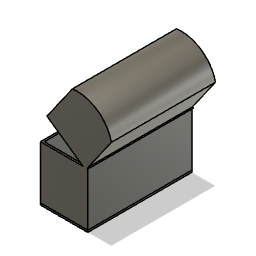
Shape 5 (Autodesk Fusion 360 design; units mm, degrees)
Autodesk Fusion 360 part; units mm, degrees
note: some values were not read from the file. Chosen so that the rebuilt part matches the saved one: which bodies a step acts on.
sketch "Sketch1" plane through (0, 0, 0) normal (0, 1, 0) x (1, 0, 0)
  line L0 (-25, 25) -> (0, 25)
  line L1 (0, 25) -> (0, -30)
  line L2 (0, -30) -> (-25, -30)
  line L3 (-25, -30) -> (-25, 25)
  constraint horizontal L0
  constraint vertical L1
  constraint horizontal L2
  constraint vertical L3
extrude "Extrude1" add sketch "Sketch1" along normal blind 50 makes body 1
sketch "Sketch2" plane through (0, 0, 0) normal (0, 0, 1) x (1, 0, 0)
  circle A0 centre (-12.3509, 42.7444) radius 18.4875
extrude "Extrude2" add sketch "Sketch2" along normal blind 30 and the other way blind 25 bodies 1
sketch "Sketch3" plane through (0, 0, 0) normal (0, 0, 1) x (1, 0, 0)
  line L0 (0, 30) -> (20, 30)
  line L1 (20, 30) -> (20, 60)
  line L2 (20, 60) -> (0, 60)
  line L3 (0, 60) -> (0, 30)
  line L4 (-25, 30) -> (-40, 30)
  line L5 (-40, 30) -> (-40, 60)
  line L6 (-40, 60) -> (-25, 60)
  line L7 (-25, 60) -> (-25, 30)
  constraint horizontal L0
  constraint vertical L1
  constraint horizontal L2
  constraint vertical L3
  constraint horizontal L4
  constraint vertical L5
  constraint horizontal L6
  constraint vertical L7
extrude "Extrude3" cut sketch "Sketch3" along normal blind 45 and the other way blind 55 bodies 1
sketch "Sketch4" plane through (0, 0, 0) normal (0, 1, 0) x (1, 0, 0)
  line L0 (-30, 25) -> (5, 25)
  line L1 (5, 25) -> (5, -35)
  line L2 (5, -35) -> (-30, -35)
  line L3 (-30, -35) -> (-30, 25)
  constraint horizontal L0
  constraint vertical L1
  constraint horizontal L2
  constraint vertical L3
extrude "Extrude4" add sketch "Sketch4" along normal blind 1 separate body makes body 2
split "Split1" by bodies 2 bodies 1 makes body 3 at (-25, 19.8411, 11.6667)
move_body "Move1" bodies 2 to x (1, 0, 0) y (0, 1, 0) z (0, 0, 1) at (0, 30, 0)
split "Split2" by bodies 2 bodies 3 makes body 4 at (-25, 19.8411, 11.6667) makes body 5 at (-23.6053, 57.4116, 11.6667)
move_body "Move2" bodies 5 to x (0.707107, -0.707107, 0) y (0.707107, 0.707107, 0) z (0, 0, 1) at (-20.9275, 9.171, 0)
shell "Shell1" thickness 1 removed faces 0 bodies 5
move_body "Move3" bodies 5 to x (1, 0, 0) y (0, 1, 0) z (0, 0, 1) at (-3.5355, -3.5355, 0)
sketch "Sketch5" plane through (0, 0, 0) normal (0, 1, 0) x (1, 0, 0)
  line L0 (-30, 25) -> (0, 25)
  line L1 (0, 25) -> (0, -35)
  line L2 (0, -35) -> (-30, -35)
  line L3 (-30, -35) -> (-30, 25)
  constraint horizontal L0
  constraint vertical L1
  constraint horizontal L2
  constraint vertical L3
shell "Shell2" thickness 1 removed faces 0 bodies 4
extrude "Extrude5" add sketch "Sketch5" along normal blind 2 separate body makes body 6
move_body "Move4" bodies 6 to x (1, 0, 0) y (0, 1, 0) z (0, 0, 1) at (0, 29, 0)
split "Split3" by bodies 6 bodies 4 makes body 7 at (-25, 19.6667, 11.6667)
move_body "Move5" bodies 5 to x (0.707107, 0.707107, 0) y (-0.707107, 0.707107, 0) z (0, 0, 1) at (64.1238, 37.9942, 0)
sketch "Sketch6" plane through (0, 0, 0) normal (0, 1, 0) x (1, 0, 0)
  line L0 (15, 30) -> (45, 30)
  line L1 (45, 30) -> (45, -35)
  line L2 (45, -35) -> (15, -35)
  line L3 (15, -35) -> (15, 30)
  constraint horizontal L0
  constraint vertical L1
  constraint horizontal L2
  constraint vertical L3
extrude "Extrude6" add sketch "Sketch6" along normal blind 1 separate body makes body 8
move_body "Move6" bodies 8 to x (1, 0, 0) y (0, 1, 0) z (0, 0, 1) at (0, 55.5, 0)
split "Split4" by bodies 8 bodies 5 makes body 9 at (25.7647, 85.2989, -6.6667)
move_body "Move7" bodies 8 to x (1, 0, 0) y (0, 1, 0) z (0, 0, 1) at (0, 1, 0)
split "Split5" by bodies 8 bodies 9 makes body 10 at (25.7647, 85.2989, -6.6667)
move_body "Move8" bodies 10 to x (0.819152, -0.573576, 0) y (0.573576, 0.819152, 0) z (0, 0, 1) at (-69.2057, 5.5064, 0)
combine "Combine1" operation add target body 10 tool bodies 7
hidden bodies 2 3 4 5 6 8 9
